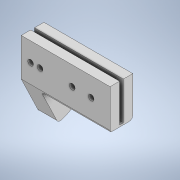
# Autodesk Inventor part: landingHolder
Saved by Autodesk Inventor 2020 (Build 240168000, 168)
## iProperties
Created: 2019-06-20
Part Number: landingHolder
Material: Generic
Document SubType Name: Modeling
Designer: Vivek Muskan
Density: 1 g/cm^3
Appearance: Default
Author: Vivek Muskan
Autodesk Inventor part; units mm, degrees
ref_plane "YZ Plane" through (0, 0, 0) normal (1, 0, 0) x (0, 1, 0)
ref_plane "XZ Plane" through (0, 0, 0) normal (0, 1, 0) x (-1, 0, 0)
sketch "Sketch1" plane through (0, 0, 0) normal (0, 0, 1) x (1, 0, 0)
  line L0 (0, 0) -> (-47, 0)
  line L1 (-47, 0) -> (-47, -20)
  line L2 (-47, -20) -> (0, -20)
  line L3 (0, -20) -> (0, 0)
  line L4 (0, 0) -> (0, -10)
  line L5 (0, -10) -> (-10, -10)
  line L6 (-10, -10) -> (-20, -10)
  line L7 (-20, -10) -> (-37, -10)
  line L8 (-37, -10) -> (-42, -10)
  circle A0 centre (-10, -10) radius 1.5
  circle A1 centre (-20, -10) radius 1.5
  circle A2 centre (-37, -10) radius 1.5
  circle A3 centre (-42, -10) radius 1.5
  dimension "d0" = 47
  dimension "d1" = 20
  dimension "d2" = 10
  dimension "d3" = 10
  dimension "d4" = 10
  dimension "d5" = 17
  dimension "d6" = 5
  dimension "d7" = 3
  dimension "d8" = 3
  dimension "d9" = 3
  dimension "d10" = 3
  constraints: 18 end point, 4 centre point, 4 coincident, 2 horizontal, 2 parallel, 2 perpendicular, 2 point on line, 1 midpoint
  measures "d0" distance of L2.end L1.end
  measures "d1" distance of L0.end L1.end
  measures "d2" distance of L0.start L4.end
  measures "d3" distance of L4.end L5.end
  measures "d4" distance of L5.end L6.end
  measures "d5" distance of L6.end L7.end
  measures "d6" distance of L7.end L8.end
  measures "d7" diameter of A0
  measures "d8" diameter of A1
  measures "d9" diameter of A2
  measures "d10" diameter of A3
extrude "Extrusion1" add sketch "Sketch1" along normal blind 5
ref_plane "Work Plane1" through (0, 0, -1) normal (0, 0, 1) x (1, 0, 0)
mirror "Mirror1" about plane through (0, 0, -1) normal (0, 0, 1) of "Extrusion1"
sketch "Sketch4" plane through (-47, -20, 0) normal (-1, 0, 0) x (0, 0, 1)
  line L0 (0, 20) -> (0, 0) projected
  line L1 (0, 0) -> (-1, 0)
  line L2 (-1, 0) -> (-16.3209, -12.8558)
  line L3 (-1, 0) -> (19, 0) construction
  line L4 (-1, 0) -> (-10.1925, -7.7135)
  line L5 (-10.1925, -7.7135) -> (-6.3623, -4.4995)
  circle A0 centre (-6.3623, -4.4995) radius 1.5
  circle A1 centre (-14.891, -6.0034) radius 1.5
  circle A2 centre (-9.3243, -12.6375) radius 1.5
  arc A3 (-21, 0) -> (-4.473, -19.6962) centre (-1, 0) ccw
  line L6 (-1, 0) -> (-4.473, -19.6962) construction
  line L7 (-1, 0) -> (-21, 0) construction
  line L8 (5, 0) -> (-4.473, -19.6962)
  line L9 (-7, 20) -> (-7, 0) projected
  line L10 (-7, 0) -> (-21, 0)
  line L11 (5, 0) -> (-21, 0)
  line L12 (-7, 0) -> (-7, -1)
  line L13 (-7, -1) -> (4.519, -1)
  line L14 (5, 0) -> (4.519, -1)
  line L15 (5, 0) -> (-7, 0)
  line L16 (-7, -1) -> (-20.975, -1)
  dimension "d27" = 1
  dimension "d28" = 20
  dimension "d29" = 140
  dimension "d30" = 12
  dimension "d31" = 5
  dimension "d32" = 3
  dimension "d35" = 360
  dimension "d37" = 20
  dimension "d38" = 80
  dimension "d42" = 1
  constraints: 30 end point, 5 horizontal, 4 centre point, 3 point on circle, 3 point on line, 2 coincident, 2 perpendicular, 1 collinear, 1 equal length, 1 vertical, 7 other
  measures "d27" distance of L0.end L1.end
  measures "d28" distance of L1.end L2.end
  measures "d29" angle of L2 L3
  measures "d30" distance of L1.end L4.end
  measures "d31" distance of L4.end L5.end
  measures "d32" diameter of A0
  measures "d37" radius of A3
  measures "d38" angle of L7 L6
  measures "d42" distance of L9.end L12.end
extrude "Extrusion2" add sketch "Sketch4" against normal blind 10 contours L11 L8 L13 L2 L1 | L2 L13 L12 L11 | L13 L8 A3 L2 A0 | L2 A0 A3 L16 L13 | L12 L16 A3 L10
extrude "Extrusion3" add sketch "Sketch4" against normal blind 47 contours L11 L8 L13 L2 L1 | L2 L13 L12 L11
extrude "Extrusion4" cut sketch "Sketch4" against normal blind 10 contours L12 L16 A3 L10
fillet "Fillet1" radius 2 2 edges at (-42, -21, -7) (-37, -21, -1.2405)
fillet "Fillet2" radius 2 2 edges at (-17.5, -21, -7) (-36.4142, -21.5858, -7)
fillet "Fillet3" radius 2 2 edges at (-42, -21, -20.975) (-42, -39.6962, -4.473)
body "Solid1"
